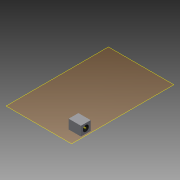
# Autodesk Inventor part: nanopc_t4_pwr
Saved by Autodesk Inventor 2013 SP2 (Build 170200200, 200)
## iProperties
Created: 2018-09-03
Part Number: nanopc_t4_pwr
Material: Generic
Document SubType Name: Modeling
Designer: alex
Density: 1 g/cm^3
Author: alex
Autodesk Inventor part; units mm, degrees
ref_plane "YZ Plane" through (0, 0, 0) normal (1, 0, 0) x (0, 1, 0)
ref_plane "XZ Plane" through (0, 0, 0) normal (0, 1, 0) x (-1, 0, 0)
ref_plane "XY Plane" through (0, 0, 0) normal (0, 0, 1) x (1, 0, 0)
ref_plane "Work Plane1" through (0, 0, 0) normal (0, 0, 1) x (1, 0, 0)
sketch "Sketch1" plane through (0, 0, 0) normal (0, 0, 1) x (1, 0, 0)
  line L0 (20.2403, -32.6932) -> (33.4403, -32.6932)
  line L1 (33.4403, -32.6932) -> (33.4403, -43.1932)
  line L2 (33.4403, -43.1932) -> (20.2403, -43.1932)
  line L3 (20.2403, -43.1932) -> (20.2403, -32.6932)
  point P0 (0, 0)
  dimension "d0" = 13.2
  dimension "d2" = 10.5
  constraints: 8 end point, 2 parallel, 1 horizontal, 1 perpendicular
  measures "d0" distance of L1.end L2.end
  measures "d2" distance of L0.end L1.end
extrude "Extrusion1" add sketch "Sketch1" along normal blind 10
sketch "Sketch2" plane through (33.4403, -43.1932, 0) normal (1, 0, 0) x (0, 0, -1)
  circle A0 centre (-5, 5.25) radius 3.25
  circle A1 centre (-5, 5.25) radius 0.75
  point P0 (0, 43.1932)
  dimension "d5" = 6.5
  dimension "d7" = 1.5
  constraints: 2 centre point, 1 coincident
  measures "d5" diameter of A0
  measures "d7" diameter of A1
extrude "Extrusion2" cut sketch "Sketch2" against normal blind 10
body "Solid1"
